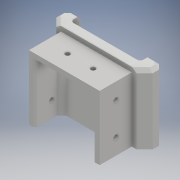
# Autodesk Inventor part: Camera mount
Saved by Autodesk Inventor 2017 (Build 210142000, 142)
## iProperties
Created: 2016-08-03
Part Number: Camera mount
Material: Generic
Document SubType Name: Modeling
Designer: Ali
Density: 1 g/cm^3
Appearance: Default
Author: Ali
Autodesk Inventor part; units mm, degrees
ref_plane "YZ Plane" through (0, 0, 0) normal (1, 0, 0) x (0, 1, 0)
ref_plane "XZ Plane" through (0, 0, 0) normal (0, 1, 0) x (-1, 0, 0)
ref_plane "XY Plane" through (0, 0, 0) normal (0, 0, 1) x (1, 0, 0)
sketch "Sketch1" plane through (0, 0, 0) normal (0, 1, 0) x (-1, 0, 0)
  line L0 (22, 20) -> (-22, 20)
  line L1 (-22, 20) -> (-22, -20)
  line L2 (-22, -20) -> (22, -20)
  line L3 (22, -20) -> (22, 20)
  line L4 (0, -20) -> (0, 20)
  line L5 (22, 0) -> (-22, 0)
  point P0 (0, 0)
  dimension "d0" = 44
  dimension "d1" = 40
  constraints: 12 end point, 6 midpoint, 2 parallel, 1 horizontal, 1 perpendicular
  measures "d0" distance of L1.end L2.end
  measures "d1" distance of L2.end L0.start
extrude "Extrusion1" add sketch "Sketch1" along normal blind 20
sketch "Sketch2" plane through (0, 20, 0) normal (0, 1, 0) x (1, 0, 0)
  line L0 (22, 20) -> (-22, 20) projected
  line L1 (-22, 20) -> (-22, -20) projected
  line L2 (-22, -20) -> (22, -20) projected
  line L3 (22, -20) -> (22, 20) projected
  line L4 (-30, -41.7016) -> (-30, 48.9081)
  line L5 (30, 51.5024) -> (30, -37.5698)
  line L6 (-22, -20) -> (22, -20) projected
  line L7 (-22, -20) -> (-30, -20)
  line L8 (-22, 20) -> (-22, -20) projected
  line L9 (-22, 20) -> (-30, 20)
  line L10 (22, -20) -> (22, 20) projected
  line L11 (22, 20) -> (30, 20)
  line L12 (22, -20) -> (30, -20)
  point P0 (0, 0)
  dimension "d4" = 30
  dimension "d5" = 30
  constraints: 12 end point, 6 point on line, 2 perpendicular, 2 vertical
  measures "d4" distance from line of L4 point (0, 0)
  measures "d5" distance from line of L5 point (0, 0)
extrude "Extrusion2" add sketch "Sketch2" along normal blind 12
sketch "Sketch3" plane through (0, 32, 0) normal (0, 1, 0) x (1, 0, 0)
  line L0 (22, 20) -> (-22, 20) projected
  line L1 (-22, -20) -> (22, -20) projected
  line L2 (-21.75, 20) -> (21.75, 20)
  line L3 (21.75, 20) -> (21.75, -20)
  line L4 (21.75, -20) -> (-21.75, -20)
  line L5 (-21.75, -20) -> (-21.75, 20)
  line L6 (-21.75, 0) -> (21.75, 0)
  point P0 (0, 0)
  dimension "d8" = 21.75
  dimension "d9" = 21.75
  constraints: 10 end point, 3 midpoint, 2 parallel, 2 point on line, 1 horizontal, 1 perpendicular
  measures "d8" distance from line of point (0, 0) L3
  measures "d9" distance from line of point (0, 0) L5
extrude "Extrusion3" cut sketch "Sketch3" against normal blind 6.5
fillet "Fillet1" radius 2 2 edges at (-21.75, 25.5, 0) (21.75, 25.5, 0)
sketch "Sketch4" plane through (-22, 0, 20) normal (0, 0, 1) x (1, 0, 0)
  line L0 (0.25, 27.5) -> (0.25, 32) projected
  line L1 (-8, 32) -> (0.25, 32) projected
  line L2 (-8, 20) -> (-8, 32) projected
  line L3 (-8, 20) -> (0, 20) projected
  line L4 (0, 0) -> (0, 20) projected
  line L5 (0, 0) -> (44, 0) projected
  line L6 (44, 0) -> (44, 20) projected
  line L7 (44, 20) -> (52, 20) projected
  line L8 (52, 20) -> (52, 32) projected
  line L9 (43.75, 32) -> (52, 32) projected
  line L10 (43.75, 32) -> (43.75, 27.5) projected
  arc A0 (41.75, 25.5) -> (43.75, 27.5) centre (41.75, 27.5) ccw projected
  line L11 (41.75, 25.5) -> (2.25, 25.5) projected
  arc A1 (0.25, 27.5) -> (2.25, 25.5) centre (2.25, 27.5) ccw projected
  line L12 (-8, 20) -> (0, 20) projected
  line L13 (0, 20) -> (44, 20)
  point P0 (22, 0)
  constraints: 2 end point, 1 collinear
extrude "Extrusion4" add sketch "Sketch4" along normal blind 3 contours A1 L11 A0 L10 L9 L8 L7 L13 L3 L2 L1 L0
chamfer "Chamfer1" distance 3 angle 45 4 edges at (25.875, 32, -20) (-25.875, 32, -20) (30, 32, 1.5) (-30, 32, 1.5)
sketch "Sketch5" plane through (22, 0, -20) normal (0, 0, -1) x (-1, 0, 0)
  line L0 (0, 0) -> (44, 0) projected
  line L1 (4, 0) -> (40, 0)
  line L2 (40, 0) -> (40, 16.2778)
  line L3 (40, 16.2778) -> (4, 16.2778)
  line L4 (4, 16.2778) -> (4, 0)
  line L5 (0, 0) -> (0, 20) projected
  line L6 (44, 0) -> (44, 20) projected
  point P0 (22, 0)
  dimension "d18" = 4
  dimension "d19" = 4
  constraints: 8 end point, 2 parallel, 1 horizontal, 1 perpendicular, 1 point on line
  measures "d18" distance between parallel lines of L4 L5
  measures "d19" distance between parallel lines of L6 L2
extrude "Extrusion5" cut sketch "Sketch5" against normal blind 36
chamfer "Chamfer2" distance 3 angle 45 3 edges at (18, 16.2778, -2) (-18, 16.2778, -2) (0, 16.2778, 16)
sketch "Sketch6" plane through (-22, 0, -20) normal (-1, 0, 0) x (0, 0, 1)
  line L0 (10, 10) -> (30, 10) construction
  line L1 (0, 0) -> (0, 20) projected
  line L2 (0, 20) -> (43, 20) projected
  point P0 (20, 0)
  dimension "d25" = 10
  dimension "d26" = 10
  dimension "d53" = 20
  constraints: 2 end point, 1 horizontal
  measures "d25" distance from line of L0.start L1
  measures "d26" distance between parallel lines of L2 L0
  measures "d53" distance of L0.end L0.start
hole "Hole1" at (-22, 10, -10) at (-22, 10, 10) direction (1, 0, 0) diameter 2.9 end through all
sketch "Sketch7" plane through (-22, 0, 20) normal (0, 0, 1) x (1, 0, 0)
  line L0 (14, 10) -> (30, 10) construction
  line L1 (-8, 20) -> (52, 20) projected
  line L2 (0, 0) -> (0, 20) projected
  point P0 (22, 0)
  dimension "d34" = 10
  dimension "d35" = 16
  dimension "d36" = 14
  constraints: 2 end point, 1 horizontal
  measures "d34" distance between parallel lines of L0 L1
  measures "d35" distance of L0.start L0.end
  measures "d36" distance from line of L2 L0.start
hole "Hole2" at (-8, 10, 20) at (8, 10, 20) direction (0, 0, -1) diameter 2.9 end through all
chamfer "Chamfer3" distance 1 angle 45 3 edges at (18, 0, -2) (0, 0, 16) (-18, 0, -2)
chamfer "Chamfer4" distance 2 angle 45 5 edges at (0, 25.5, -20) (21.1642, 26.0858, -20) (21.75, 28.25, -20) (-21.1642, 26.0858, -20) (-21.75, 28.25, -20)
chamfer "Chamfer5" distance 5 angle 45 2 edges at (30, 20, 1.5) (-30, 20, 1.5)
chamfer "Chamfer6" distance 2 angle 45 8 edges at (-27.5, 22.5, 23) (-30, 27, 23) (-28.5, 30.5, 23) (-24.375, 32, 23) (27.5, 22.5, 23) (30, 27, 23) (28.5, 30.5, 23) (24.375, 32, 23)
sketch "Sketch8" plane through (0, 25.5, 0) normal (0, 1, 0) x (1, 0, 0)
  line L0 (19.75, 20) -> (-19.75, 20) projected
  point P0 (0, 0)
  point P1 (0, -7)
  dimension "d57" = 27
  measures "d57" distance from line of L0 point (0, -7)
hole "Hole3" at (0, 25.5, 7) direction (0, -1, 0) diameter 6.2 end through all
sketch "Sketch9" plane through (-15, 16.2778, -20) normal (0, -1, 0) x (1, 0, 0)
  circle A0 centre (15, 27) radius 3.1 projected
  circle A1 centre (15, 27) radius 5.9
  point P0 (15, 20)
  dimension "d65" = 2.8
  constraints: 1 centre point
  measures "d65" radial gap between concentric circles of A0 A1
extrude "Extrusion6" cut sketch "Sketch9" against normal blind 1.2
equation "\"d9\" = d8"
body "Solid1"
